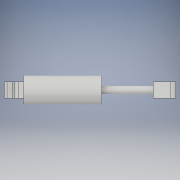
# Autodesk Inventor part: amortiguador
Saved by Autodesk Inventor 2018 (Build 220112000, 112)
## iProperties
Created: 2017-04-25
Part Number: amortiguador
Material: Generic
Document SubType Name: Modeling
Designer: eroldan
Density: 1 g/cm^3
Appearance: Default
Author: eroldan
Autodesk Inventor part; units mm, degrees
ref_plane "YZ Plane" through (0, 0, 0) normal (1, 0, 0) x (0, 1, 0)
ref_plane "XZ Plane" through (0, 0, 0) normal (0, 1, 0) x (-1, 0, 0)
ref_plane "XY Plane" through (0, 0, 0) normal (0, 0, 1) x (1, 0, 0)
sketch "Sketch12" plane through (0, 0, 0) normal (0, 0, 1) x (1, 0, 0)
  line L0 (120.2458, -10.6408) -> (144.8251, -10.6408)
  line L1 (152.8251, -2.6408) -> (152.8251, 2.6408)
  line L2 (144.8251, 10.6408) -> (120.2458, 10.6408)
  arc A0 (144.8251, -10.6408) -> (152.8251, -2.6408) centre (144.8251, -2.6408) ccw
  arc A1 (152.8251, 2.6408) -> (144.8251, 10.6408) centre (144.8251, 2.6408) ccw
  circle A2 centre (146.8251, 0) radius 4
  circle A3 centre (-93.1749, 0) radius 4 construction
  line L3 (120.2458, -10.6408) -> (120.2458, 10.6408)
  line L4 (-83.9681, -12.6932) -> (-87.2761, -6.1075)
  line L5 (-87.2761, -6.1075) -> (-95.1749, -6.1075)
  line L6 (-87.2761, 6.1075) -> (-95.1749, 6.1075)
  circle A4 centre (-93.1749, 0) radius 4
  arc A5 (-95.1749, 6.1075) -> (-99.1749, 2.1075) centre (-95.1749, 2.1075) ccw
  line L7 (-99.1749, 2.1075) -> (-99.1749, 0)
  arc A6 (-99.1749, -2.1075) -> (-95.1749, -6.1075) centre (-95.1749, -2.1075) ccw
  line L8 (-99.1749, -2.1075) -> (-99.1749, 0)
  arc A7 (-83.9681, -12.6932) -> (-78.6065, -16) centre (-78.6065, -10) ccw
  line L9 (-71, -16) -> (-78.6065, -16)
  line L10 (-71, 0) -> (-71, -16)
  line L11 (-71, 20) -> (-71, -20)
  line L12 (-83.9681, 12.6932) -> (-87.2761, 6.1075)
  line L13 (-71, 0) -> (-71, 16)
  line L14 (-71, 16) -> (-78.6065, 16)
  arc A8 (-78.6065, 16) -> (-83.9681, 12.6932) centre (-78.6065, 10) ccw
  point P0 (0, 0)
  dimension "d44" = 8
  dimension "d45" = 8
  dimension "d46" = 240
  dimension "d47" = 6
  dimension "d48" = 6
  dimension "d49" = 16
  dimension "d50" = 4
  dimension "d51" = 8
  dimension "d52" = 6
  constraints: 30 end point, 12 point on circle, 9 centre point, 8 tangent, 3 perpendicular, 2 parallel, 1 equal radius, 1 horizontal, 1 midpoint, 1 vertical
  measures "d44" radius of A0
  measures "d45" diameter of A2
  measures "d46" distance of A2.centre A3.centre
  measures "d47" distance from line of L1 A2.centre
  measures "d48" radius of A7
  measures "d49" distance of L10.start L9.start
  measures "d50" radius of A6
  measures "d51" diameter of A4
  measures "d52" distance of L7.end A4.centre
extrude "Extrusion14" add sketch "Sketch12" along normal blind 24 contours L4 L5 A6 L8 L7 A5 L6 L12 A8 L14 L11 L10 L9 A7
sketch "Sketch14" plane through (-71, -16, 0) normal (1, 0, 0) x (0, 0, -1)
  line L0 (0, 0) -> (-24, 0) projected
  line L1 (-24, 12) -> (-24, 20) projected
  circle A0 centre (-12, 16) radius 19
  circle A1 centre (-12, 16) radius 21
  point P0 (0, 16)
  dimension "d58" = 38
  dimension "d59" = 2
  constraints: 2 centre point
  measures "d58" diameter of A0
  measures "d59" radial gap between concentric circles of A0 A1
extrude "Extrusion16" add sketch "Sketch14" along normal blind 115
sketch "Sketch15" plane through (-71, 0, 12) normal (-1, 0, 0) x (0, 0, 1)
  circle A0 centre (0, 0) radius 21 projected
  point P0 (-12, 0)
extrude "Extrusion17" add sketch "Sketch15" against normal blind 4
sketch "Sketch16" plane through (44, 0, 12) normal (1, 0, 0) x (0, 0, -1)
  circle A0 centre (0, 0) radius 21 projected
  point P0 (12, 0)
extrude "Extrusion18" add sketch "Sketch16" against normal blind 4
sketch "Sketch17" plane through (0, 0, 0) normal (0, 0, 1) x (1, 0, 0)
  line L0 (120, -10.6408) -> (144.8251, -10.6408)
  line L1 (152.8251, -2.6408) -> (152.8251, 2.6408)
  line L2 (144.8251, 10.6408) -> (120, 10.6408)
  arc A0 (144.8251, -10.6408) -> (152.8251, -2.6408) centre (144.8251, -2.6408) ccw
  arc A1 (152.8251, 2.6408) -> (144.8251, 10.6408) centre (144.8251, 2.6408) ccw
  circle A2 centre (146.8251, 0) radius 4
  line L3 (120, -10.6408) -> (120, 10.6408)
  line L4 (44, -21) -> (44, 21) projected
  point P0 (0, 0)
  point P1 (0, 0)
  dimension "d68" = 8
  dimension "d69" = 8
  dimension "d71" = 6
  dimension "d77" = 76
  constraints: 8 end point, 4 point on circle, 4 tangent, 3 centre point, 2 perpendicular, 1 equal radius, 1 horizontal, 1 parallel
  measures "d68" radius of A0
  measures "d69" diameter of A2
  measures "d71" distance from line of L1 A2.centre
  measures "d77" distance between parallel lines of L3 L4
extrude "Extrusion20" add sketch "Sketch17" along normal blind 24 separate body
sketch "Sketch18" plane through (120, -10.6408, 0) normal (-1, 0, 0) x (0, 0, 1)
  line L0 (0, 0) -> (24, 0) projected
  circle A0 centre (12, 10.6408) radius 6
  point P0 (0, 10.6408)
  point P1 (0, 12.7482)
  dimension "d80" = 12
  constraints: 1 centre point, 1 coincident
  measures "d80" diameter of A0
extrude "Extrusion21" add sketch "Sketch18" along normal up to surface (76 mm away) bodies 2
